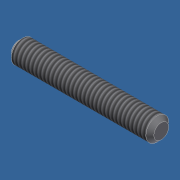
# Autodesk Inventor part: BN425_M4x25
Saved by Autodesk Inventor 2021.2 (Build 252289000, 289)
## iProperties
Created: 2021-06-20
Part Number: BN425_M4x25
Material: Acier zingué-bleu
Description: Goujons filetés
Document SubType Name: Modeling
Designer: Jean-Marc.VULLIAMY
Authority: B&R 861478
Density: 1.4 g/cm^3
Appearance: Par défaut
Mass: 0.432208 g
Surface Area: 3.27711 cm^2
Volume: 0.30872 cm^3
Material number: ---
Author: Jean-Marc.VULLIAMY
Autodesk Inventor part; units mm, degrees
ref_plane "Plan YZ" through (0, 0, 0) normal (1, 0, 0) x (0, 1, 0)
ref_plane "Plan XZ" through (0, 0, 0) normal (0, 1, 0) x (-1, 0, 0)
ref_plane "Plan XY" through (0, 0, 0) normal (0, 0, 1) x (1, 0, 0)
sketch "Esquisse1" plane through (0, 0, 0) normal (0, 0, 1) x (1, 0, 0)
  line L0 (0, 0) -> (25, 0)
  line L1 (25, 0) -> (25, 2)
  line L2 (25, 2) -> (0, 2)
  line L3 (0, 2) -> (0, 0)
  line L4 (-5, 0) -> (30, 0) construction
  dimension "d0" = 4
  dimension "d1" = 25
  constraints: 8 end point, 2 parallel, 1 horizontal, 1 perpendicular
  measures "d0" diameter of L2 L4
  measures "d1" distance of L1.end L2.end
revolve "Révolution1" add sketch "Esquisse1" angle 360 about axis through (-10, 0, 0) along (1, 0, 0)
thread "Filetage1" size "M4x0.7" designation "M4" class "6g" standard "ISO M" full length
chamfer "Chanfrein1" distance 0.7 angle 45 2 edges at (25, -2, 0) (0, -2, 0)
